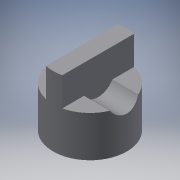
# Autodesk Inventor part: PistonCylinder
Saved by Autodesk Inventor 2016 (Build 200138000, 138)
## iProperties
Created: 2017-02-18
Part Number: PistonCylinder
Material: Generic
Document SubType Name: Modeling
Designer: Owner
Density: 1 g/cm^3
Appearance: Default
Author: Owner
Autodesk Inventor part; units mm, degrees
ref_plane "YZ Plane" through (0, 0, 0) normal (1, 0, 0) x (0, 1, 0)
ref_plane "XZ Plane" through (0, 0, 0) normal (0, 1, 0) x (-1, 0, 0)
ref_plane "XY Plane" through (0, 0, 0) normal (0, 0, 1) x (1, 0, 0)
sketch "Sketch1" plane through (0, 0, 0) normal (0, 1, 0) x (-1, 0, 0)
  circle A0 centre (0, 0) radius 4.5
  dimension "d0" = 9
  constraints: 1 centre point, 1 coincident
  measures "d0" diameter of A0
extrude "Extrusion1" add sketch "Sketch1" along normal blind 5
sketch "Sketch2" plane through (0, 5, 0) normal (0, 1, 0) x (1, 0, 0)
  circle A0 centre (0, 0) radius 4.5 projected
  line L0 (0, 0) -> (-1, 0)
  line L1 (-1, 0) -> (1, 0)
  line L2 (1, 0) -> (1, 8.5977)
  line L3 (1, 8.5977) -> (-1, 8.5977)
  line L4 (-1, 8.5977) -> (-1, -7.4697)
  line L5 (-1, -7.4697) -> (1, -7.4697)
  line L6 (1, -7.4697) -> (1, 8.5977)
  dimension "d4" = 1
  dimension "d5" = 2
  constraints: 14 end point, 4 perpendicular, 2 point on line, 1 collinear, 1 horizontal
  measures "d4" distance of L0.start L0.end
  measures "d5" distance of L0.end L1.end
extrude "Extrusion2" add sketch "Sketch2" along normal blind 5 contours L2 L1 L0 L4 A0 | A0 L4 L3 L2 | L6 L5 L4 A0 | A0 L4 L0 L1 L6
sketch "Sketch3" plane through (0, 5, 0) normal (0, -1, 0) x (1, 0, 0)
  arc A0 (1, 4.3875) -> (-1, 4.3875) centre (0, 0) ccw projected
  line L0 (1, 7.4697) -> (1, 4.3875) projected
  line L1 (-1, 7.4697) -> (1, 7.4697) projected
  line L2 (-1, 4.3875) -> (-1, 7.4697) projected
  arc A1 (-1, -4.3875) -> (1, -4.3875) centre (0, 0) ccw projected
  line L3 (-1, -8.5977) -> (-1, -4.3875) projected
  line L4 (1, -8.5977) -> (-1, -8.5977) projected
  line L5 (1, -4.3875) -> (1, -8.5977) projected
extrude "Extrusion3" cut sketch "Sketch3" against normal blind 5
sketch "Sketch7" plane through (1, 5, 4.3875) normal (1, 0, 0) x (0, 0, -1)
  line L0 (4.3875, 2) -> (4.3875, 1)
  circle A0 centre (4.3875, 1) radius 2
  point P0 (4.3875, -5)
  dimension "d20" = 1
  dimension "d21" = 4
  constraints: 2 end point, 1 centre point, 1 coincident, 1 vertical
  measures "d20" distance of L0.start L0.end
  measures "d21" diameter of A0
extrude "Extrusion7" cut sketch "Sketch7" along normal blind 25.4
sketch "Sketch8" plane through (1, 5, -4.3875) normal (1, 0, 0) x (0, 0, -1)
  line L0 (0, 5) -> (-8.775, 5) projected
  line L1 (0, 5) -> (-8.775, 5)
  line L2 (-8.775, 5) -> (-10.2746, 5)
  line L3 (-10.2746, 5) -> (-10.2746, 3.5)
  line L4 (-10.2746, 3.5) -> (1.1183, 3.5)
  line L5 (1.1183, 3.5) -> (1.1183, 5)
  line L6 (1.1183, 5) -> (0, 5)
  point P0 (-4.3875, -5)
  dimension "d24" = 1.5
  constraints: 12 end point, 3 perpendicular, 2 horizontal, 1 point on line
  measures "d24" distance of L2.end L3.end
extrude "Extrusion8" cut sketch "Sketch8" against normal blind 25.4
fillet "Fillet2" radius 1 2 edges at (0, 8.5, 4.5) (0, 8.5, -4.5)
body "Solid1"
